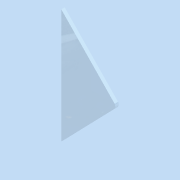
# Autodesk Inventor part: 본체 창 2
Saved by Autodesk Inventor 2020 (Build 240168000, 168)
## iProperties
Created: 2020-05-05
Part Number: 본체 창 2
Material: 일반
Document SubType Name: Modeling
Designer: sbahn
Density: 1 g/cm^3
Appearance: 선명
Author: sbahn
Autodesk Inventor part; units mm, degrees
ref_plane "YZ Plane" through (0, 0, 0) normal (1, 0, 0) x (0, 1, 0)
ref_plane "XZ Plane" through (0, 0, 0) normal (0, 1, 0) x (-1, 0, 0)
ref_plane "XY Plane" through (0, 0, 0) normal (0, 0, 1) x (1, 0, 0)
sketch "스케치1" plane through (0, 0, 0) normal (0, 0, 1) x (1, 0, 0)
  line L0 (-8.6981, -1.3757) -> (-39.2674, -32.97) projected
  line L1 (-39.2674, -32.97) -> (-39.2674, 33) projected
  arc A0 (-8.6981, -1.3757) -> (-8.6981, 1.4057) centre (-10.1355, 0.015) ccw projected
  line L2 (-39.2674, 33) -> (-8.6981, 1.4057)
  point P0 (0, 0)
  point P1 (-8.6981, 1.4057)
  constraints: 2 end point
extrude "돌출1" add sketch "스케치1" against normal blind 2
